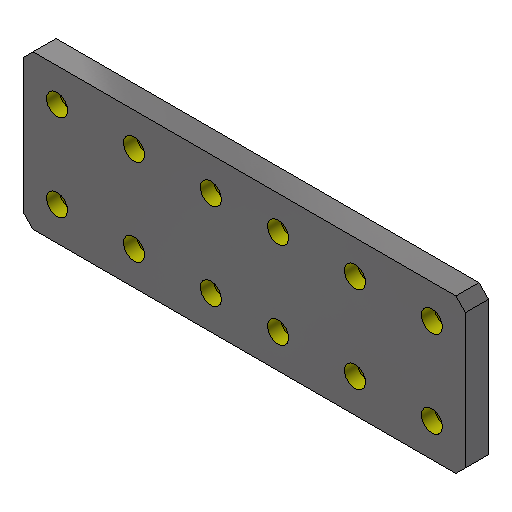
# Autodesk Inventor part: TL20240701-10100CV-001
Saved by Autodesk Inventor 2022.5 (Build 265521000, 521)
## iProperties
Category: PROFILE ASSY
Company: 현대 트랜시스
Created: 2023-04-03
Part Number: TL20240701-10100CV-001
Checked By: 김형민
Engr Approved By: 김시현
User Status: 2 x48
Material: SS400
Description: 0
Document SubType Name: Modeling
Mfg Approved By: 호상태
Designer: 김형민
Stock Number: 001
Density: 7.85 g/cm^3
Appearance: Plating Zinc White
Project: TL20240701
DETAIL: Coveryor Assembly
M/C TITLE: CJ 제일제당 협동로봇 포장시스탬 PILOT 장비
PARTS NAME: Bracket
SPECIFICATION: TA20221101-CV200000-015
DocNumber: 221118_Standard_v1
Folder: .\
VDS_Category: 엔지니어링
Detail Description: Processed products
Title: PROFILE BRACKET
Subject: SW차종 시트조립라인
Author: 박성규
Revision Number: A
Autodesk Inventor part; units mm, degrees
ref_plane "YZ Plane" through (0, 0, 0) normal (1, 0, 0) x (0, 1, 0)
ref_plane "XZ Plane" through (0, 0, 0) normal (0, 1, 0) x (-1, 0, 0)
ref_plane "XY Plane" through (0, 0, 0) normal (0, 0, 1) x (1, 0, 0)
sketch "스케치9" plane through (0, 0, 0) normal (0, 0, 1) x (1, 0, 0)
  line L0 (-20, 40) -> (20, 40)
  line L1 (20, 40) -> (20, -40)
  line L2 (20, -40) -> (-20, -40)
  line L3 (-20, -40) -> (-20, 40)
  line L4 (-20, 40) -> (20, -40) construction
  line L5 (20, 40) -> (-20, -40) construction
  line L6 (-20, 28) -> (8, 28)
  line L7 (8, 40) -> (8, -40)
  line L8 (8, -40) -> (-20, -40)
  line L9 (-20, -40) -> (-20, 28)
  point P0 (0, 0)
  dimension "d40" = 40
  dimension "d41" = 80
  dimension "d42" = 12
  dimension "d43" = 12
  constraints: 20 end point, 4 parallel, 4 point on line, 2 horizontal, 2 midpoint, 2 perpendicular
  measures "d40" distance of L0.start L0.end
  measures "d41" distance of L0.end L1.end
  measures "d42" distance between parallel lines of L1 L7
  measures "d43" distance between parallel lines of L0 L6
extrude "돌출4" add sketch "스케치9" along normal mid plane 230 contours L0 L1 L2 L7
sketch "스케치13" plane through (8, 30, 115) normal (-1, 0, 0) x (0, 1, 0)
  line L0 (-7.5, 132.5) -> (-52.5, 132.5)
  line L1 (-52.5, 132.5) -> (-52.5, 212.5)
  line L2 (-52.5, 212.5) -> (-7.5, 212.5)
  line L3 (-7.5, 212.5) -> (-7.5, 132.5)
  line L4 (-7.5, 132.5) -> (-52.5, 212.5) construction
  line L5 (-52.5, 132.5) -> (-7.5, 212.5) construction
  line L6 (10, 230) -> (10, 0) projected
  line L7 (10, 115) -> (-70, 115) construction
  line L8 (-70, 230) -> (-70, 0) projected
  line L9 (-7.5, 97.5) -> (-52.5, 97.5)
  line L10 (-52.5, 97.5) -> (-52.5, 17.5)
  line L11 (-52.5, 17.5) -> (-7.5, 17.5)
  line L12 (-7.5, 17.5) -> (-7.5, 97.5)
  line L13 (-7.5, 97.5) -> (-52.5, 17.5) construction
  line L14 (-52.5, 97.5) -> (-7.5, 17.5) construction
  point P0 (-30, 172.5)
  point P1 (-30, 172.5)
  point P2 (-30, 172.5)
  point P3 (-30, 172.5)
  point P4 (-30, 115)
  point P5 (-30, 57.5)
  point P6 (-30, 57.5)
  point P7 (-30, 57.5)
  point P8 (-30, 57.5)
  point P9 (-52.5, 172.5)
  point P10 (-7.5, 172.5)
  point P11 (-52.5, 57.5)
  point P12 (-7.5, 57.5)
  dimension "d74" = 80
  dimension "d75" = 45
  dimension "d103" = 35
  dimension "d104" = 17.5
  constraints: 26 end point, 13 midpoint, 8 symmetric about line, 3 coincident, 2 parallel, 1 horizontal, 1 perpendicular, 1 vertical alignment
  measures "d74" distance of L0.end L1.end
  measures "d75" distance of L1.end L2.end
  measures "d103" diameter of L0 L7
  measures "d104" distance between parallel lines of L8 L1
hole "구멍6" at (8, 22.5, -17.5) at (8, 22.5, -97.5) at (8, -22.5, -97.5) at (8, -22.5, -17.5) at (8, 22.5, 97.5) at (8, -22.5, 97.5) at (8, -22.5, 17.5) at (8, 22.5, 17.5) at (8, 22.5, -57.5) at (8, -22.5, -57.5) at (8, -22.5, 57.5) at (8, 22.5, 57.5) direction (1, 0, 0) diameter 6.6 end through all counterbore diameter 11 counterbore depth 6.8 clearance for "Socket Head Cap Screw ISO 4762" size "M6" standard "ISO"
chamfer "모따기1" distance 5 angle 45 4 edges at (14, 40, -115) (14, -40, -115) (14, 40, 115) (14, -40, 115)
fillet "모깎기7" [suppressed]
equation "\"d43\" = d42"
